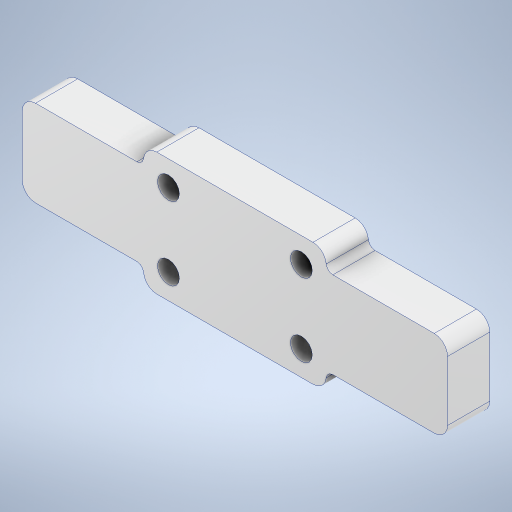
# Autodesk Inventor part: Printhead Belt Retainer Cap THICK
Saved by Autodesk Inventor 2024 (Build 280153000, 153)
## iProperties
Created: 2025-01-04
Part Number: Printhead Belt Retainer Cap THICK
Material: Aluminum 6061
Document SubType Name: Modeling
Designer: Ishaan
Density: 2.7 g/cm^3
Appearance: Aluminum - Flat
Author: Ishaan
Autodesk Inventor part; units mm, degrees
ref_plane "YZ Plane" through (0, 0, 0) normal (1, 0, 0) x (0, 1, 0)
ref_plane "XZ Plane" through (0, 0, 0) normal (0, 1, 0) x (-1, 0, 0)
ref_plane "XY Plane" through (0, 0, 0) normal (0, 0, 1) x (1, 0, 0)
sketch "Sketch1" plane through (0, 0, 0) normal (0, 0, 1) x (1, 0, 0)
  line L0 (13.75, -9.25) -> (-13.75, -9.25)
  line L1 (-13.75, -9.25) -> (-13.75, 9.25)
  line L2 (-13.75, 9.25) -> (13.75, 9.25)
  line L3 (13.75, 9.25) -> (13.75, -9.25)
  line L4 (13.75, -9.25) -> (-13.75, 9.25) construction
  line L5 (-13.75, -9.25) -> (13.75, 9.25) construction
  line L6 (-18, 0) -> (18, 0) construction
  circle A0 centre (-18, 0) radius 4
  circle A1 centre (18, 0) radius 4
  line L7 (32, -1) -> (-32, -1)
  line L8 (-32, -1) -> (-32, 1)
  line L9 (-32, 1) -> (32, 1)
  line L10 (32, 1) -> (32, -1)
  line L11 (32, -1) -> (-32, 1) construction
  line L12 (-32, -1) -> (32, 1) construction
  line L13 (32, -6.5) -> (-32, -6.5)
  line L14 (-32, -6.5) -> (-32, 6.5)
  line L15 (-32, 6.5) -> (32, 6.5)
  line L16 (32, 6.5) -> (32, -6.5)
  line L17 (32, -6.5) -> (-32, 6.5) construction
  line L18 (-32, -6.5) -> (32, 6.5) construction
  point P0 (0, 0)
  point P1 (-21.873, -1)
  point P2 (-13.75, -6.5)
  point P3 (13.75, -6.5)
  point P4 (21.873, -1)
  point P5 (21.873, 1)
  point P6 (13.75, 6.5)
  point P7 (-13.75, 6.5)
  point P8 (-21.873, 1)
  dimension "d0" = 27.5
  dimension "d1" = 18.5
  dimension "d2" = 8
  dimension "d3" = 8
  dimension "d4" = 36
  dimension "d5" = 64
  dimension "d6" = 2
  dimension "d7" = 13
  constraints: 38 end point, 7 midpoint, 6 parallel, 4 horizontal, 3 perpendicular, 2 centre point, 2 coincident, 1 collinear
  measures "d0" distance of L1.end L2.end
  measures "d1" distance of L0.end L1.end
  measures "d2" diameter of A0
  measures "d3" diameter of A1
  measures "d4" distance of L6.start L6.end
  measures "d5" distance of L8.end L9.end
  measures "d6" distance between parallel lines of L7 L9
  measures "d7" distance of L13.end L14.end
extrude "Extrusion1" add sketch "Sketch1" along normal blind 6.35
fillet "Fillet1" radius 2 4 edges at (13.75, 9.25, 3.175) (-13.75, 9.25, 3.175) (-13.75, -9.25, 3.175) (13.75, -9.25, 3.175)
fillet "Fillet2" radius 2 4 edges at (-32, 6.5, 3.175) (-32, -6.5, 3.175) (32, 6.5, 3.175) (32, -6.5, 3.175)
fillet "Fillet3" radius 1 4 edges at (-13.75, -6.5, 3.175) (-13.75, 6.5, 3.175) (13.75, 6.5, 3.175) (13.75, -6.5, 3.175)
sketch "Sketch2" plane through (0, 0, 6.35) normal (0, 0, 1) x (1, 0, 0)
  line L0 (10, -5.5) -> (-10, -5.5) construction
  line L1 (-10, -5.5) -> (-10, 5.5) construction
  line L2 (-10, 5.5) -> (10, 5.5) construction
  line L3 (10, 5.5) -> (10, -5.5) construction
  line L4 (10, -5.5) -> (-10, 5.5) construction
  line L5 (-10, -5.5) -> (10, 5.5) construction
  circle A0 centre (-10, 5.5) radius 3 construction
  circle A1 centre (-10, -5.5) radius 3 construction
  circle A2 centre (-10, 5.5) radius 1.65 construction
  line L6 (11.75, 9.25) -> (-11.75, 9.25) construction
  point P0 (0, 0)
  dimension "d13" = 20
  dimension "d14" = 11
  dimension "d22" = 6
  dimension "d23" = 6
  dimension "d25" = 3.3
  dimension "d26" = 2.1
  constraints: 12 end point, 7 coincident, 3 centre point, 2 midpoint, 2 parallel, 1 horizontal, 1 perpendicular
  measures "d13" distance of L1.end L2.end
  measures "d14" distance of L0.end L1.end
  measures "d22" diameter of A0
  measures "d23" diameter of A1
  measures "d25" diameter of A2
  measures "d26" distance edge to line of A2 L6
hole "Hole1" at (-10, 5.5, 6.35) at (10, 5.5, 6.35) at (10, -5.5, 6.35) at (-10, -5.5, 6.35) direction (0, 0, -1) diameter 3.3 end through all
body "Solid1"
